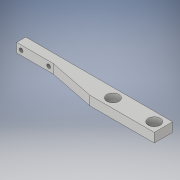
# Autodesk Inventor part: WheelSuspensionFork
Saved by Autodesk Inventor 2017 (Build 210142000, 142)
## iProperties
Created: 2018-05-09
Part Number: WheelSuspensionFork
Material: Generic
Document SubType Name: Modeling
Designer: User
Density: 1 g/cm^3
Appearance: Default
Author: User
Autodesk Inventor part; units mm, degrees
ref_plane "YZ Plane" through (0, 0, 0) normal (1, 0, 0) x (0, 1, 0)
ref_plane "XZ Plane" through (0, 0, 0) normal (0, 1, 0) x (-1, 0, 0)
ref_plane "XY Plane" through (0, 0, 0) normal (0, 0, 1) x (1, 0, 0)
sketch "Sketch1" plane through (0, 0, 0) normal (0, 1, 0) x (-1, 0, 0)
  line L0 (0, 0) -> (101.6, 0)
  line L1 (0, -12.7) -> (44.45, -12.7)
  line L2 (44.45, -12.7) -> (76.2, -12.7)
  line L3 (44.45, 0) -> (76.2, -6.35)
  line L4 (76.2, -6.35) -> (101.6, -6.35)
  line L5 (76.2, -12.7) -> (101.6, -12.7)
  line L6 (0, -12.7) -> (0, 0)
  line L7 (101.6, -12.7) -> (101.6, -6.35)
  point P0 (101.6, -6.35)
  dimension "d5" = 44.45
  dimension "d6" = 12.7
  dimension "d7" = 44.45
  dimension "d16" = 6.35
  dimension "d55" = 6.35
  dimension "d58" = 31.75
  dimension "d59" = 101.6
  constraints: 16 end point, 2 horizontal, 2 vertical, 1 point on line
  measures "d5" distance of L1.start L1.end
  measures "d6" distance between parallel lines of L0 L1
  measures "d7" distance of L0.start L3.start
  measures "d16" distance between parallel lines of L0 L4
  measures "d55" distance between parallel lines of L4 L5
  measures "d58" horizontal distance of L3.start L3.end
  measures "d59" distance between parallel lines of L6 L7
extrude "Extrusion2" add sketch "Sketch1" along normal blind 6.35
sketch "Sketch5" plane through (0, 6.35, 0) normal (0, 1, 0) x (1, 0, 0)
  line L0 (-44.45, 0) -> (0, 0) projected
  line L1 (0, 0) -> (0, 12.7) projected
  line L2 (0, 12.7) -> (-101.6, 12.7) projected
  line L3 (-101.6, 12.7) -> (-101.6, 6.35) projected
  line L4 (-101.6, 6.35) -> (-76.2, 6.35) projected
  line L5 (-76.2, 6.35) -> (-44.45, 0) projected
  point P0 (-6.35, 6.35)
  point P1 (-34.925, 6.35)
  dimension "d60" = 6.35
  dimension "d61" = 6.35
  dimension "d62" = 6.35
  dimension "d63" = 28.575
  dimension "d64" = 12.7
  measures "d60" distance from line of point (-6.35, 6.35) L2
  measures "d61" distance from line of L1 point (-6.35, 6.35)
  measures "d62" distance from line of L2 point (-34.925, 6.35)
  measures "d63" distance of point (-6.35, 6.35) point (-34.925, 6.35)
  measures "d64" distance of L0.end L1.end
hole "Hole4" at (-6.35, 6.35, -6.35) at (-34.925, 6.35, -6.35) direction (0, -1, 0) diameter 8.382 depth 25.4 tip angle 118
sketch "Sketch6" plane through (-101.6, 0, -6.35) normal (0, 0, 1) x (1, 0, 0)
  line L0 (25.4, 0) -> (0, 0) projected
  line L1 (25.4, 0) -> (25.4, 6.35) projected
  line L2 (0, 6.35) -> (25.4, 6.35) projected
  line L3 (0, 0) -> (0, 6.35) projected
  point P0 (101.6, 0)
  point P1 (3.175, 3.175)
  point P2 (22.225, 3.175)
  dimension "d72" = 6.35
  dimension "d73" = 3.175
  dimension "d74" = 3.175
  dimension "d75" = 19.05
  dimension "d76" = 3.175
  measures "d72" distance of L0.end L2.start
  measures "d73" distance from line of L2 point (3.175, 3.175)
  measures "d74" distance from line of point (22.225, 3.175) L2
  measures "d75" distance of point (22.225, 3.175) point (3.175, 3.175)
  measures "d76" distance from line of L3 point (3.175, 3.175)
hole "Hole5" at (-98.425, 3.175, -6.35) at (-79.375, 3.175, -6.35) direction (0, 0, -1) diameter 2.6416 depth 10.9728 tip angle 118 thread size "6-32 UNC" class "2B" standard "ANSI Unified Screw Threads"
equation "\"d5\" = d10"
equation "\"d7\" = d5"
equation "\"d60\" = 0.5 * d64"
equation "\"d61\" = d60"
equation "\"d62\" = d60"
equation "\"d73\" = 0.5 * d72"
equation "\"d74\" = d73"
equation "\"d76\" = d73"
equation "\"d10\" = 44.45"
body "Solid1"
